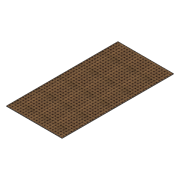
# Autodesk Inventor part: Tepih
Saved by Autodesk Inventor 2020.2 (Build 242310000, 310)
## iProperties
Created: 2020-10-18
Part Number: Tepih
Material: Carpet
Document SubType Name: Modeling
Designer: User
Density: 0.19 g/cm^3
Appearance: Light Brown - Dark Brown Squares
Author: User
Autodesk Inventor part; units mm, degrees
ref_plane "YZ Plane" through (0, 0, 0) normal (1, 0, 0) x (0, 1, 0)
ref_plane "XZ Plane" through (0, 0, 0) normal (0, 1, 0) x (-1, 0, 0)
ref_plane "XY Plane" through (0, 0, 0) normal (0, 0, 1) x (1, 0, 0)
sketch "Sketch1" plane through (0, 0, 0) normal (0, 1, 0) x (-1, 0, 0)
  line L0 (-354, 888) -> (646, 888)
  line L1 (646, 888) -> (646, -1112)
  line L2 (646, -1112) -> (-354, -1112)
  line L3 (-354, -1112) -> (-354, 888)
  point P0 (0, 0)
  dimension "d0" = 1000
  dimension "d1" = 2000
  constraints: 8 end point, 2 parallel, 1 horizontal, 1 perpendicular
  measures "d0" distance of L1.end L2.end
  measures "d1" distance of L0.end L1.end
extrude "Extrusion1" add sketch "Sketch1" along normal blind 5
body "Solid1"
